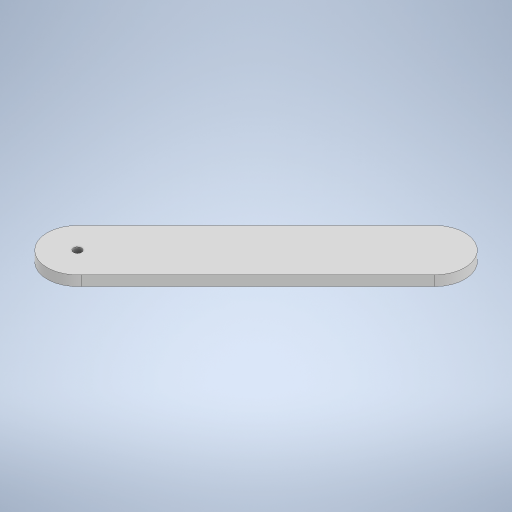
# Autodesk Inventor part: Бедро
Saved by Autodesk Inventor 2023.2 (Build 272271000, 271)
## iProperties
Created: 2024-07-30
Part Number: Бедро
Material: Типовые
Document SubType Name: Modeling
Designer: End_Ways
Density: 1 g/cm^3
Appearance: По умолчанию
Author: End_Ways
Autodesk Inventor part; units mm, degrees
ref_plane "YZ Plane" through (0, 0, 0) normal (1, 0, 0) x (0, 1, 0)
ref_plane "XZ Plane" through (0, 0, 0) normal (0, 1, 0) x (-1, 0, 0)
ref_plane "XY Plane" through (0, 0, 0) normal (0, 0, 1) x (1, 0, 0)
sketch "Эскиз1" plane through (0, 0, 0) normal (0, 1, 0) x (-1, 0, 0)
  circle A0 centre (0, 0) radius 30
  circle A1 centre (0, 0) radius 4
  line L0 (0, 0) -> (-176.7767, -176.7767)
  line L1 (0, 0) -> (250, 0) construction
  circle A2 centre (-176.7767, -176.7767) radius 30
  line L2 (-22.9528, 19.3176) -> (-197.9804, -155.554)
  line L3 (20.2164, -22.1652) -> (-155.5608, -197.9872)
  point P0 (-206.64, -173.9156)
  point P1 (18.7548, -23.4149)
  dimension "d0" = 60
  dimension "d1" = 8
  dimension "d2" = 250
  dimension "d3" = 135
  dimension "d4" = 60
  constraints: 8 end point, 6 point on circle, 3 centre point, 3 coincident, 2 tangent, 1 equal length, 1 horizontal
  measures "d0" diameter of A0
  measures "d1" diameter of A1
  measures "d2" distance of L0.start L0.end
  measures "d3" angle of L0 L1
  measures "d4" diameter of A2
extrude "Выдавливание1" add sketch "Эскиз1" along normal blind 10
